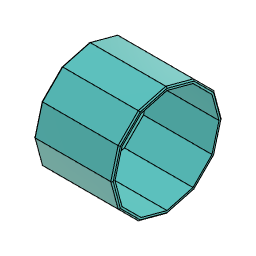
Switch_End_Cap (Autodesk Fusion 360 design; units mm, degrees)
Autodesk Fusion 360 part; units mm, degrees
sketch "Hexagonal Surface" plane through (0, 0, 0) normal (1, 0, 0) x (0, 1, 0)
  line L0 (-22, 0) -> (-19.0526, -11)
  line L1 (-19.0526, -11) -> (-11, -19.0526)
  line L2 (-11, -19.0526) -> (0, -22)
  line L3 (0, -22) -> (11, -19.0526)
  line L4 (11, -19.0526) -> (19.0526, -11)
  line L5 (19.0526, -11) -> (22, 0)
  line L6 (22, 0) -> (19.0526, 11)
  line L7 (19.0526, 11) -> (11, 19.0526)
  line L8 (11, 19.0526) -> (0, 22)
  line L9 (0, 22) -> (-11, 19.0526)
  line L10 (-11, 19.0526) -> (-19.0526, 11)
  line L11 (-19.0526, 11) -> (-22, 0)
  line L12 (-11.647, -20.1733) -> (0, -23.2941)
  line L13 (0, -23.2941) -> (11.647, -20.1733)
  line L14 (11.647, -20.1733) -> (20.1733, -11.647)
  line L15 (20.1733, -11.647) -> (23.2941, 0)
  line L16 (23.2941, 0) -> (20.1733, 11.647)
  line L17 (20.1733, 11.647) -> (11.647, 20.1733)
  line L18 (11.647, 20.1733) -> (0, 23.2941)
  line L19 (0, 23.2941) -> (-11.647, 20.1733)
  line L20 (-11.647, 20.1733) -> (-20.1733, 11.647)
  line L21 (-20.1733, 11.647) -> (-23.2941, 0)
  line L22 (-23.2941, 0) -> (-20.1733, -11.647)
  line L23 (-20.1733, -11.647) -> (-11.647, -20.1733)
  dimension "d1" = 22
  dimension "d2" = 1.25
  measures "d1" distance of L0.start origin
extrude "Extrude1" add sketch "Hexagonal Surface" along normal blind 4 contours L0 L1 L2 L3 L4 L5 L6 L7 L8 L9 L10 L11 | L12 L13 L14 L15 L16 L17 L18 L19 L20 L21 L22 L23
extrude "Extrude2" add sketch "Hexagonal Surface" along normal blind 29 from surface at 4
fillet "Rounded Edges" radius 0.5 12 edges at (0, 15.9102, -15.9102) (0, 5.8235, -21.7337) (0, -5.8235, -21.7337) (0, -15.9102, -15.9102) (0, -21.7337, -5.8235) (0, -21.7337, 5.8235) (0, -15.9102, 15.9102) (0, -5.8235, 21.7337) (0, 5.8235, 21.7337) (0, 15.9102, 15.9102) (0, 21.7337, 5.8235) (0, 21.7337, -5.8235)
fillet "Rounded Edges" radius 0.5 12 edges at (33, 5.8235, 21.7337) (33, -5.8235, 21.7337) (33, -15.9102, 15.9102) (33, -21.7337, 5.8235) (33, -21.7337, -5.8235) (33, -15.9102, -15.9102) (33, -5.8235, -21.7337) (33, 5.8235, -21.7337) (33, 15.9102, -15.9102) (33, 21.7337, -5.8235) (33, 21.7337, 5.8235) (33, 15.9102, 15.9102)
sketch "Switch and Buttons Access" plane through (0, 0, 0) normal (-1, 0, 0) x (0, -1, 0)
  line L0 (11.3882, -19.725) -> (19.725, -11.3882)
  line L1 (19.725, -11.3882) -> (22.7765, 0)
  line L2 (22.7765, 0) -> (19.725, 11.3882)
  line L3 (19.725, 11.3882) -> (11.3882, 19.725)
  line L4 (11.3882, 19.725) -> (0, 22.7765)
  line L5 (0, 22.7765) -> (-11.3882, 19.725)
  line L6 (-11.3882, 19.725) -> (-19.725, 11.3882)
  line L7 (-19.725, 11.3882) -> (-22.7765, 0)
  line L8 (-22.7765, 0) -> (-19.725, -11.3882)
  line L9 (-19.725, -11.3882) -> (-11.3882, -19.725)
  line L10 (-11.3882, -19.725) -> (0, -22.7765)
  line L11 (0, -22.7765) -> (11.3882, -19.725)
  line L12 (-14, -1.4) -> (14, -1.4)
  arc A0 (14, -1.4) -> (14, 6.6) centre (14, 2.6) ccw
  line L13 (14, 6.6) -> (-14, 6.6)
  arc A1 (-14, 6.6) -> (-14, -1.4) centre (-14, 2.6) ccw
  line L14 (-14, 2.6) -> (14, 2.6) construction
  line L15 (-14, -3.0693) -> (14, -3.0693)
  arc A2 (14, -3.0693) -> (14, 8.2693) centre (14, 2.6) ccw
  line L16 (14, 8.2693) -> (-14, 8.2693)
  arc A3 (-14, 8.2693) -> (-14, -3.0693) centre (-14, 2.6) ccw
  dimension "d12" = 4
  dimension "d13" = 28
  dimension "d15" = 1.6693
  dimension "d29" = 14
  dimension "d30" = 6.6
  constraint tangent L12 A0
  constraint tangent A0 L13
  constraint parallel L12 L13
  constraint tangent L13 A1
  constraint tangent L12 A1
  constraint horizontal L14
  measures "d12" radius of A1
  measures "d13" distance of A0.end L13.end
  measures "d29" horizontal distance of origin A1.centre
  measures "d30" distance of origin L13
extrude "Extrude8" cut sketch "Switch and Buttons Access" against normal through all contours L12 A0 L13 A1
chamfer "Buttons Access Chamfer" distance 2 angle 45 4 edges at (0, 0, -1.4) (0, 18, 2.6) (0, 0, 6.6) (0, -18, 2.6)
sketch "Labels" plane through (0, 0, 0) normal (-1, 0, 0) x (0, -1, 0)
  line L0 (11.3882, -19.725) -> (19.725, -11.3882)
  line L1 (19.725, -11.3882) -> (22.7765, 0)
  line L2 (22.7765, 0) -> (19.725, 11.3882)
  line L3 (19.725, 11.3882) -> (11.3882, 19.725)
  line L4 (11.3882, 19.725) -> (0, 22.7765)
  line L5 (0, 22.7765) -> (-11.3882, 19.725)
  line L6 (-11.3882, 19.725) -> (-19.725, 11.3882)
  line L7 (-19.725, 11.3882) -> (-22.7765, 0)
  line L8 (-22.7765, 0) -> (-19.725, -11.3882)
  line L9 (-19.725, -11.3882) -> (-11.3882, -19.725)
  line L10 (-11.3882, -19.725) -> (0, -22.7765)
  line L11 (0, -22.7765) -> (11.3882, -19.725)
  line L12 (-15.1556, -6.1595) -> (-2.815, -6.2154) construction
  line L13 (-2.815, -6.2154) -> (-2.815, -6.2139) construction
  line L14 (-2.815, -6.2139) -> (-15.1556, -6.158) construction
  line L15 (-15.1556, -6.158) -> (-15.1556, -6.1595) construction
  line L16 (-7.6132, 9.3386) -> (1.9842, 9.3386) construction
  line L17 (1.9842, 9.3386) -> (1.9842, 12.9725) construction
  line L18 (1.9842, 12.9725) -> (-7.6132, 12.9725) construction
  line L19 (-7.6132, 12.9725) -> (-7.6132, 9.3386) construction
  line L20 (7.8642, -9.6526) -> (19.0039, -9.6526) construction
  line L21 (19.0039, -9.6526) -> (19.0039, -6.0186) construction
  line L22 (19.0039, -6.0186) -> (7.8642, -6.0186) construction
  line L23 (7.8642, -6.0186) -> (7.8642, -9.6526) construction
  line L24 (14, -3.4) -> (-14, -3.4)
  arc A0 (-14, 8.6) -> (-14, -3.4) centre (-14, 2.6) ccw
  line L25 (-14, 8.6) -> (14, 8.6)
  arc A1 (14, -3.4) -> (14, 8.6) centre (14, 2.6) ccw
  dimension "d24" = 3
  dimension "d25" = 3
  dimension "d26" = 3
  text T0 "VOL" font "Arial" height 3 align left top in box 12.3407 x 0.0015 at (-15.1556, -6.1595) x (0.99999, -0.004534) y (0.004534, 0.99999) spacing 1
  text T1 "ON/OFF" font "Arial" height 3 align left top in box 9.5974 x 3.6339 at (-7.6132, 9.3386) x (1, 0) y (0, 1) spacing 1
  text T2 "SKIP" font "Arial" height 3 align left top in box 11.1398 x 3.6339 at (7.8642, -9.6526) x (1, 0) y (0, 1) spacing 1
extrude "Label Cutouts" cut sketch "Labels" against normal blind 1 text T0 T2 T1
named bodies: "Switch End Cap"
